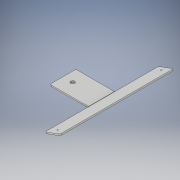
# Autodesk Inventor part: Top Mount
Saved by Autodesk Inventor 2019 (Build 230136000, 136)
## iProperties
Created: 2020-02-21
Part Number: Top Mount
Material: Generic
Document SubType Name: Sheet Metal
Designer: gfb14170
Density: 1 g/cm^3
Sheet Metal Rule: Default_mm
Appearance: Default
Author: gfb14170
Autodesk Inventor part; units mm, degrees
ref_plane "YZ Plane" through (0, 0, 0) normal (1, 0, 0) x (0, 1, 0)
ref_plane "XZ Plane" through (0, 0, 0) normal (0, 1, 0) x (-1, 0, 0)
ref_plane "XY Plane" through (0, 0, 0) normal (0, 0, 1) x (1, 0, 0)
sketch "Sketch1" plane through (0, 0, 0) normal (0, 1, 0) x (-1, 0, 0)
  line L0 (30, 20) -> (-30, 20)
  line L1 (-30, 20) -> (-30, -20)
  line L2 (-30, -20) -> (30, -20)
  line L3 (30, -20) -> (30, 20)
  point P0 (0, 0)
  dimension "d0" = 20
  dimension "d1" = 20
  dimension "d2" = 30
  dimension "d3" = 30
  measures "d0" distance from line of point (0, 0) L0
  measures "d1" distance from line of point (0, 0) L2
  measures "d2" distance from line of point (0, 0) L3
  measures "d3" distance from line of point (0, 0) L1
extrude "Plate1" add sketch "Sketch1" along normal blind 2
sketch "Sketch3" plane through (29.316, 1.8794, -20) normal (0.3420201, -0.9396926, 0) x (0.9396926, 0.3420201, 0)
  line L0 (0, 40) -> (0, 0)
  line L1 (0, 0) -> (25, 0)
  line L2 (25, 0) -> (25, 40)
  line L3 (25, 40) -> (0, 40)
  constraints: 6 end point, 1 horizontal, 1 perpendicular, 1 vertical
edge flange "Flange1" height 25 angle 20 thickness 2 bend radius 2 thickness toward (0.3420201, -0.9396926, 0) relief straight relief width 2 relief depth 1 edges at (30, 2, 0) wall of the first edge with corners at (29.316, 1.8794, 20) (29.316, 1.8794, -20) (52.8083, 10.4299, -20) (52.8083, 10.4299, 20)
bend "Bend1"
corner "Corner1"
sketch "Sketch4" plane through (52.8083, 10.4299, 20) normal (-0.3420201, 0.9396926, 0) x (0.9396926, 0.3420201, 0)
  line L0 (-24.2947, 40) -> (-24.2947, 0) projected
  line L1 (-24.2947, 0) -> (0, 0) projected
  line L2 (0, 0) -> (0, 40) projected
  line L3 (-24.2947, 40) -> (0, 40) projected
  line L4 (-24.2947, -67.5) -> (0, -67.5)
  line L5 (0, -67.5) -> (0, 107.5)
  line L6 (0, 107.5) -> (-24.2947, 107.5)
  line L7 (-24.2947, 107.5) -> (-24.2947, -67.5)
  point P0 (-53.1908, 20)
  dimension "d19" = 67.5
  dimension "d20" = 67.5
  dimension "d21" = 0
  dimension "d22" = 0
  constraints: 8 end point, 2 parallel, 1 horizontal, 1 perpendicular
  measures "d19" distance between parallel lines of L4 L1
  measures "d20" distance between parallel lines of L6 L3
  measures "d21" distance between parallel lines of L2 L5
  measures "d22" distance between parallel lines of L0 L7
extrude "Extrusion1" add sketch "Sketch4" against normal blind 2 contours L7 L6 L5 L3 | L1 L5 L4 L7
fillet "Fillet1" radius 2 2 edges at (-30, 1, 20) (-30, 1, -20)
fillet "Fillet2" radius 2 4 edges at (30.3208, 1.1809, 87.5) (53.1503, 9.4902, 87.5) (53.1503, 9.4902, -87.5) (30.3208, 1.1809, -87.5)
sketch "Sketch5" plane through (0, 2, 0) normal (0, 1, 0) x (1, 0, 0)
  circle A0 centre (-15, 0) radius 3
  point P0 (0, 0)
  dimension "d27" = 6
  dimension "d28" = 15
  dimension "d29" = 0
  constraints: 1 centre point
  measures "d27" diameter of A0
  measures "d28" distance of A0.centre point (0, 0)
  measures "d29" vertical distance of point (0, 0) A0.centre
extrude "Extrusion2" cut sketch "Sketch5" against normal blind 2
sketch "Sketch6" plane through (29.9787, 2.1206, 20) normal (-0.3420201, 0.9396926, 0) x (0.9396926, 0.3420201, 0)
  circle A0 centre (12, -59.5) radius 1
  arc A1 (2, 107.5) -> (0, 105.5) centre (2, 105.5) ccw projected
  line L0 (0, 105.5) -> (0, 40) projected
  line L1 (0, 40) -> (0, 0) projected
  line L2 (0, 0) -> (0, -65.5) projected
  arc A2 (0, -65.5) -> (2, -67.5) centre (2, -65.5) ccw projected
  line L3 (2, -67.5) -> (22.2947, -67.5) projected
  arc A3 (22.2947, -67.5) -> (24.2947, -65.5) centre (22.2947, -65.5) ccw projected
  line L4 (24.2947, -65.5) -> (24.2947, 105.5) projected
  arc A4 (24.2947, 105.5) -> (22.2947, 107.5) centre (22.2947, 105.5) ccw projected
  line L5 (22.2947, 107.5) -> (2, 107.5) projected
  circle A5 centre (12, 100.5) radius 1
  point P0 (-28.8961, 20)
  dimension "d32" = 2
  dimension "d35" = 160
  dimension "d40" = 8
  dimension "d41" = 12
  constraints: 2 centre point, 1 vertical, 2 other
  measures "d32" diameter of A0
  measures "d35" distance of A0.centre A5.centre
  measures "d40" distance from line of L3 A0.centre
  measures "d41" distance from line of L2 A0.centre
extrude "Extrusion3" cut sketch "Sketch6" against normal blind 2 contours A0 | A5
equation "\"d20\" = d19"
equation "\"d1\" = d0"
equation "\"BendRadius\" = Thickness"
equation "\"BendReliefWidth\" = Thickness"
equation "\"BendReliefDepth\" = 0.5 * Thickness"
equation "\"CornerReliefSize\" = 4 * Thickness"
equation "\"MinimumRemnant\" = 2 * Thickness"
equation "\"TransitionRadius\" = BendRadius"
equation "\"JacobiRadiusSize\" = BendRadius"
equation "\"GapSize\" = Thickness"
body "Solid1"
